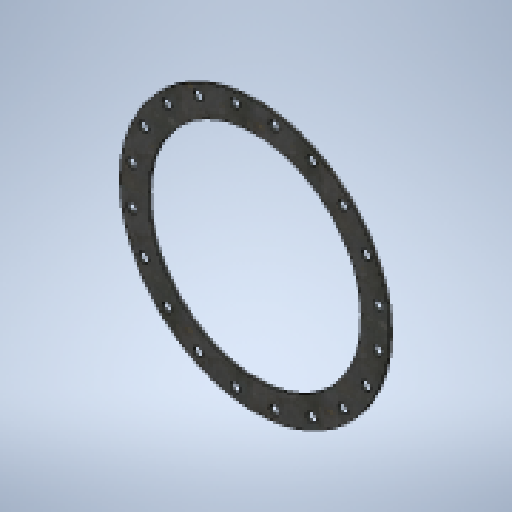
# Autodesk Inventor part: ANP 1403 accses hatch flange
Saved by Autodesk Inventor 2025 (Build 290162010, 162A)
## iProperties
Created: 2025-02-12
Part Number: ANP 1403 accses hatch flange
Material: Steel
Document SubType Name: Sheet Metal
Designer: pokla
Density: 7.85 g/cm^3
Flat Pattern Width: 67 cm
Flat Pattern Length: 67 cm
Flat Pattern Area: 4489 cm^2
Sheet Metal Rule: Default_mm
Sheet Metal Width: 670,000 mm
Sheet Metal Length: 670,000 mm
Sheet Metal Area: 448900,000 mm^2
Appearance: Plate
Author: pokla
Autodesk Inventor part; units mm, degrees
ref_plane "YZ Plane" through (0, 0, 0) normal (1, 0, 0) x (0, 1, 0)
ref_plane "XZ Plane" through (0, 0, 0) normal (0, 1, 0) x (-1, 0, 0)
ref_plane "XY Plane" through (0, 0, 0) normal (0, 0, 1) x (1, 0, 0)
sketch "Sketch1" plane through (0, 0, 0) normal (0, 1, 0) x (-1, 0, 0)
  circle A0 centre (0, 0) radius 265
  circle A1 centre (0, 0) radius 335
  line L0 (335, 0) -> (265, 0)
  line L1 (-265, 0) -> (-335, 0)
  line L2 (0, 265) -> (0, 335)
  point P0 (300, 0)
  point P1 (-300, 0)
  point P2 (0, 300)
  dimension "d1" = 670
  dimension "d4" = 530
  constraints: 6 end point, 6 point on circle, 3 midpoint, 2 centre point, 2 coincident, 2 horizontal, 2 horizontal alignment, 1 vertical, 1 vertical alignment
  measures "d1" diameter of A1
  measures "d4" diameter of A0
extrude "Extrusion1" add sketch "Sketch1" along normal blind 6 contours L0 A1 L1 A0 | A0 L2 A1 L0 | A0 L1 A1 L2
sketch "Sketch2" plane through (0, 0, 0) normal (0, -1, 0) x (1, 0, 0)
  circle A0 centre (0, 0) radius 335 projected
  circle A1 centre (0, 0) radius 265 projected
  circle A2 centre (48.4947, 306.1834) radius 11.5
  circle A3 centre (0, 0) radius 265 projected
  line L0 (48.4947, 306.1834) -> (0, 0)
  point P0 (0, 265)
  point P1 (265, 0)
  dimension "d5" = 310
  dimension "d7" = 23
  constraints: 2 end point, 1 centre point
  measures "d5" distance of point (0, 0) L0.start
  measures "d7" diameter of A2
extrude "Cut1" cut sketch "Sketch2" against normal blind 6 contours A2
pattern_circular "Circular Pattern1" count 20 over 360 about axis through (0, 0, 0) along (0, 1, 0) of "Cut1"
equation "\"d9\" = Thickness"
equation "\"BendRadius\" = Thickness"
equation "\"BendReliefWidth\" = Thickness"
equation "\"BendReliefDepth\" = 0.5 * Thickness"
equation "\"CornerReliefSize\" = 4 * Thickness"
equation "\"MinimumRemnant\" = 2 * Thickness"
equation "\"TransitionRadius\" = BendRadius"
equation "\"JacobiRadiusSize\" = BendRadius"
equation "\"GapSize\" = Thickness"
equation "\"d8\" = Thickness"
equation "\"Thickness\" = 6"
body "Solid1"
